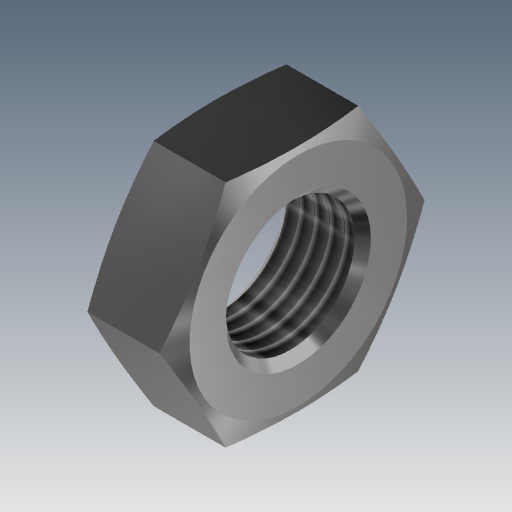
# Autodesk Inventor part: C96S40_NUT
Saved by Autodesk Inventor 2021 (Build 250183000, 183)
## iProperties
Part Number: C96S40_NUT
Material: Stainless Steel, Polished
Catalog Web Link: www.cadenas.de
Description: C96 NUT-ISO Cylinder:Standard Double Acting,Single/Double Rod
Vendor: SMC
Document SubType Name: Modeling
Designer: partserver
Manufacturer: SMC
Mass: 12.245 g
Surface Area: 10.8544 cm^2
Volume: 1.53063 cm^3
Density: 8 g/cm^3
Appearance: Stainless - Polished
Category: PARTsolutions
Company: SMC
PSOL_IDENT_0: {$CADENAS_DATA\23d-libs\smc_jp\actuator\standard_air_cylinder\cp96_c96\c96\parts\c96_nut.prj},174 {V
PSOL_IDENT_1: TYP=3D},{NB=C96S40_NUT},{LINA=C96S40_NUT},{NN=C96 NUT},{DATE=18.06.2021 10:30:46},{GEOMDATE=23.04.20
PSOL_IDENT_2: 12 00:00:00},{VERSION=v090415094912},{LINEID=60},{WBVAR=},{WBNUMERIC=}  {NB=C96S40_NUT},{LINA=C96S40
PSOL_IDENT_3: _NUT},{KT=DUMMY},{BORE=40},{KK=M12x1.25},{KRA=12},{KRP=1.25},{H=7},{B=19}
NB: C96S40_NUT
NN: C96 NUT
NT: ISO Cylinder:Standard Double Acting,Single/Double Rod
NBSYN: C96S$BORE._NUT
LINA: C96S40_NUT
CATALOG: SMC (JP
BORE: 40
KK: M12x1.25
H: 7
B: 19
SUPPLIER: SMC
ARTICLENO: C96S40_NUT
BOMINFO: C96S40_NUT
CREATOR: CADENAS GmbH
Title: C96S40_NUT
Author: Cadenas PARTsolutions
Comments: ISO Cylinder:Standard Double Acting,Single/Double Rod
Autodesk Inventor part; units mm, degrees
sketch "Sketch_2" plane through (0, 0, 0) normal (0, 0, 1) x (1, 0, 0)
  line L0 (3.5, 0) -> (-3.5, 0)
  line L1 (-3.5, 9) -> (-3.5, 6)
  line L2 (-3.5, 6) -> (-2.8235, 5.3235)
  line L3 (-2.8235, 5.3235) -> (2.8235, 5.3235)
  line L4 (2.8235, 5.3235) -> (3.5, 6)
  line L5 (3.5, 6) -> (3.5, 9)
  line L6 (3.5, 9) -> (2.3478, 13.3)
  line L7 (2.3478, 13.3) -> (-2.3478, 13.3)
  line L8 (-2.3478, 13.3) -> (-3.5, 9)
  constraints: 18 end point
revolve "Revolution1" add sketch "Sketch_2" angle 360 about axis through (3.5, 0, 0) along (1, 0, 0)
thread "Thread1" size "M12x1.25" class "6H" standard "ISO Metric profile" full length
sketch "Sketch_3" plane through (0, 0, 0) normal (1, 0, 0) x (0, 1, 0)
  circle A0 centre (0, 0) radius 19
  line L0 (-5.4848, 9.5) -> (-10.9697, 0)
  line L1 (-10.9697, 0) -> (-5.4848, -9.5)
  line L2 (-5.4848, -9.5) -> (5.4848, -9.5)
  line L3 (5.4848, -9.5) -> (10.9697, 0)
  line L4 (10.9697, 0) -> (5.4848, 9.5)
  line L5 (5.4848, 9.5) -> (-5.4848, 9.5)
  constraints: 12 end point, 1 centre point
extrude "Extrusion1" cut sketch "Sketch_3" along normal mid plane 7
ref_plane "NUT_ROD_XY" through (0, 0, 0) normal (1, 0, 0) x (0, 0, -1)
ref_plane "NUT_ROD_YZ" through (0, 0, 0) normal (0, 0, -1) x (0, 1, 0)
ref_plane "NUT_ROD_ZX" through (0, 0, 0) normal (0, 1, 0) x (1, 0, 0)
body "Solid1"
